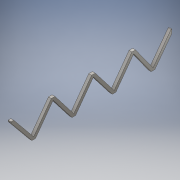
# Autodesk Inventor part: Truss Structure
Saved by Autodesk Inventor 2016 (Build 200138000, 138)
## iProperties
Created: 2019-03-24
Part Number: Truss Structure
Material: Stainless Steel
Document SubType Name: Modeling
Designer: benja
Density: 8 g/cm^3
Appearance: Semi-Polished
Author: benja
Autodesk Inventor part; units mm, degrees
ref_plane "YZ Plane" through (0, 0, 0) normal (1, 0, 0) x (0, 1, 0)
ref_plane "XZ Plane" through (0, 0, 0) normal (0, 1, 0) x (-1, 0, 0)
ref_plane "XY Plane" through (0, 0, 0) normal (0, 0, 1) x (1, 0, 0)
sketch "Sketch1" plane through (0, 0, 0) normal (1, 0, 0) x (0, 1, 0)
  line L0 (937.5, 0) -> (972.5, 0)
  line L1 (142.4751, -1299.6011) -> (-32.2024, -1299.6011)
  line L2 (-799.6982, 0) -> (-972.5, 0)
  line L3 (-972.5, 0) -> (-32.2024, -1299.6011)
  line L4 (-799.6982, 0) -> (55.5287, -1182.0234)
  line L5 (-2760.5427, 0) -> (-2937.5, 0)
  line L6 (-972.5, 0) -> (-1928.1041, -1305.6863)
  line L7 (-886.2529, -119.2036) -> (-1754.6144, -1305.6863)
  line L8 (-1754.6144, -1305.6863) -> (-1928.1041, -1305.6863)
  line L9 (-1928.1041, -1305.6863) -> (-2937.5, 0)
  line L10 (-1842.0475, -1188.1032) -> (-2760.5427, 0)
  line L11 (-2937.5, 0) -> (-3893.1041, -1305.6863)
  line L12 (-2848.3805, -115.2789) -> (-3719.6144, -1305.6863)
  line L13 (-3893.1041, -1305.6863) -> (-4902.5, 0)
  line L14 (-3717.928, -1303.3821) -> (-4725.5427, 0)
  line L15 (-4902.5, 0) -> (-5848.2043, -1300)
  line L16 (-4813.306, -115.3753) -> (-5675.0789, -1300)
  line L17 (-3719.6144, -1305.6863) -> (-3893.1041, -1305.6863)
  line L18 (-5675.0789, -1300) -> (-5848.2043, -1300)
  line L19 (142.4751, -1299.6011) -> (972.5, -187.1966)
  line L20 (-32.2024, -1299.6011) -> (937.5, 0)
  line L21 (972.5, 0) -> (972.5, -187.1966)
  line L22 (-6867.5, 0) -> (-6736.369, 0)
  line L23 (-6867.5, -60.967) -> (-5848.2043, -1300)
  line L24 (-6736.369, 0) -> (-5763.1277, -1183.0505)
  line L25 (-6867.5, 0) -> (-6867.5, -60.967)
  line L26 (-4725.5427, 0) -> (-4902.5, 0)
  line L27 (142.4751, -1299.6011) -> (-6414.4595, -1299.6011)
  line L28 (-4902.5, 0) -> (-4052.5, 0) construction
  point P0 (0, 0)
  point P1 (-3807.0475, -1188.1032)
  point P2 (-5806.9041, -1243.2271)
  dimension "d0" = 972.5
  dimension "d1" = 1300
  dimension "d5" = 972.5
  dimension "d6" = 140
  dimension "d7" = 1965
  dimension "d8" = 140
  dimension "d9" = 140
  dimension "d10" = 1965
  dimension "d11" = 140
  dimension "d12" = 140
  dimension "d13" = 1965
  dimension "d14" = 140
  dimension "d24" = 35
  dimension "d27" = 140
  dimension "d32" = 140
  constraints: 58 end point, 12 point on line, 11 horizontal, 8 parallel, 2 vertical
  measures "d0" distance of point (0, 0) L0.end
  measures "d1" distance of point (0, 0) L1.end
  measures "d5" distance of point (0, 0) L2.end
  measures "d6" distance between parallel lines of L3 L4
  measures "d7" distance of L2.end L5.end
  measures "d8" distance between parallel lines of L7 L6
  measures "d9" distance between parallel lines of L9 L10
  measures "d10" distance of L5.end L13.end
  measures "d11" distance between parallel lines of L12 L11
  measures "d12" distance between parallel lines of L13 L14
  measures "d13" distance of L13.end L22.start
  measures "d14" distance between parallel lines of L16 L15
  measures "d24" distance of L0.start L0.end
  measures "d27" distance between parallel lines of L24 L23
  measures "d32" distance between parallel lines of L19 L20
extrude "Extrusion2" add sketch "Sketch1" along normal blind 140 contours L0 L21 L19 L1 L20 | L20 L3 L2 L4 | L3 L7 L27 L6 | L7 L8 L6 L27 | L6 L27 L9 L5 L10 | L6 L9 L27 | L9 L12 L27 L14 L11 | L12 L14 L27 | L14 L27 L11 | L11 L27 L13 L26 L14 | L12 L17 L11 L27 L14 | L11 L13 L27 | L13 L16 L27 L15 | L16 L18 L15 L27 | L15 L27 L23 L25 L22 L24 | L15 L23 L27
body "Solid2"
